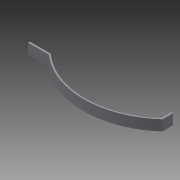
# Autodesk Inventor part: RearSkidSteel
Saved by Autodesk Inventor 2014 (Build 180170000, 170)
## iProperties
Created: 2016-02-11
Part Number: RearSkidSteel
Material: Generic
Document SubType Name: Modeling
Designer: choices
Density: 1 g/cm^3
Appearance: Default
Author: choices
Autodesk Inventor part; units mm, degrees
ref_plane "YZ Plane" through (0, 0, 0) normal (1, 0, 0) x (0, 1, 0)
ref_plane "XZ Plane" through (0, 0, 0) normal (0, 1, 0) x (-1, 0, 0)
ref_plane "XY Plane" through (0, 0, 0) normal (0, 0, 1) x (1, 0, 0)
sketch "Sketch1" plane through (0, 0, 0) normal (1, 0, 0) x (0, 1, 0)
  line L0 (-19.6181, -6.8872) -> (-0.5681, -6.8872)
  line L1 (-0.5681, -6.8872) -> (-0.5681, -10.0622)
  line L2 (-0.5681, -10.0622) -> (-19.6181, -10.0622)
  line L3 (-19.6181, -10.0622) -> (-19.6181, -6.8872)
  dimension "d7" = 19.05
  dimension "d8" = 3.175
  constraints: 8 end point, 2 parallel, 1 horizontal, 1 perpendicular
  measures "d7" distance of L1.end L2.end
  measures "d8" distance of L0.end L1.end
extrude "Extrusion1" add sketch "Sketch1" along normal blind 38.1
sketch "Sketch2" plane through (0, -0.5681, -6.8872) normal (0, 1, 0) x (1, 0, 0)
  line L0 (38.1, 3.175) -> (38.1, 0) projected
  arc A0 (38.1, 1.5875) -> (241.3, 1.5875) centre (139.7, 115.1798) ccw
  line L1 (0, 0) -> (38.1, 0) projected
  point P0 (0, -6.8872)
  dimension "d11" = 203.2
  dimension "d12" = 152.4
  dimension "d17" = 1.5875
  constraints: 2 point on circle, 1 centre point, 1 midpoint
  measures "d11" distance of A0.start A0.end
  measures "d12" radius of A0
  measures "d17" distance from line of A0.end L1
sketch "Sketch3" plane through (38.1, 0, 0) normal (1, 0, 0) x (0, 0, -1)
  line L0 (6.8872, -0.5681) -> (6.8872, -19.6181) projected
  line L1 (6.8872, -19.6181) -> (10.0622, -19.6181) projected
  line L2 (10.0622, -19.6181) -> (10.0622, -0.5681) projected
  line L3 (10.0622, -0.5681) -> (6.8872, -0.5681) projected
  point P0 (0, 0)
sweep "Sweep1" add profiles "Sketch3" path "Sketch2" path curves A0
sketch "Sketch4" plane through (0, -0.5681, -6.8872) normal (0, 1, 0) x (1, 0, 0)
  line L0 (239.7223, 1.7639) -> (242.8777, 1.4111) projected
  line L1 (0, 3.175) -> (38.1, 3.175) projected
  line L2 (239.7223, 1.7639) -> (239.7223, 20.8139)
  line L3 (239.7223, 20.8139) -> (242.8777, 20.8139)
  line L4 (242.8777, 20.8139) -> (242.8777, 1.4111)
  point P0 (0, -6.8872)
  dimension "d14" = 19.05
  constraints: 6 end point, 2 perpendicular, 1 parallel
  measures "d14" distance of L0.start L2.end
extrude "Extrusion2" add sketch "Sketch4" against normal blind 19.05
body "Solid1"
